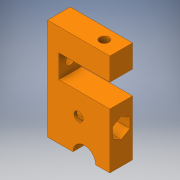
# Autodesk Inventor part: vexOverSupportForArm
Saved by Autodesk Inventor 2016 SP1 (Build 200210100, 210)
## iProperties
Created: 2015-08-15
Part Number: vexOverSupportForArm
Material: Generic
Document SubType Name: Modeling
Designer: steele
Density: 1 g/cm^3
Appearance: Orange
Author: steele
Autodesk Inventor part; units mm, degrees
note: some values were not read from the file. Chosen so that the rebuilt part matches the saved one: direction of "Hole8".
ref_plane "YZ Plane" through (0, 0, 0) normal (1, 0, 0) x (0, 1, 0)
ref_plane "XZ Plane" through (0, 0, 0) normal (0, 1, 0) x (-1, 0, 0)
ref_plane "XY Plane" through (0, 0, 0) normal (0, 0, 1) x (1, 0, 0)
sketch "Sketch1" plane through (0, 0, 0) normal (0, 0, 1) x (1, 0, 0)
  line L0 (0, 0) -> (-34.798, 0)
  line L1 (-34.798, 0) -> (-34.798, -56.642)
  line L2 (0, -12.7) -> (-28.448, -12.7)
  line L3 (-28.448, -12.7) -> (-28.448, -25.654)
  line L4 (-28.448, -25.654) -> (0, -25.654)
  line L5 (0, -56.642) -> (0, -25.654)
  line L6 (0, -12.7) -> (0, 0)
  arc A0 (-7.874, -56.642) -> (-20.574, -56.642) centre (-14.224, -56.642) ccw
  line L7 (-34.798, -56.642) -> (-20.574, -56.642)
  line L8 (-7.874, -56.642) -> (0, -56.642)
  dimension "d0" = 56.642
  dimension "d1" = 34.798
  dimension "d4" = 12.7
  dimension "d5" = 28.448
  dimension "d6" = 12.954
  dimension "d50" = 6.35
  dimension "d51" = 14.224
  dimension "d71" = 56.642
  dimension "d72" = 56.642
  constraints: 18 end point, 4 parallel, 2 horizontal, 2 perpendicular, 2 point on circle, 1 centre point, 1 collinear
  measures "d0" distance of L0.end L1.end
  measures "d1" distance of L0.start L0.end
  measures "d4" distance between parallel lines of L2 L0
  measures "d5" distance of L2.start L2.end
  measures "d6" distance between parallel lines of L4 L2
  measures "d50" radius of A0
  measures "d51" distance from line of A0.centre L5
  measures "d71" distance from line of L0 A0.centre
  measures "d72" distance between parallel lines of L0 L8
extrude "Extrusion4" add sketch "Sketch1" along normal mid plane 12.7
sketch "Sketch9" plane through (-34.798, -56.642, 6.35) normal (-1, 0, 0) x (0, 0, 1)
  line L0 (-12.7, 30.988) -> (0, 30.988) construction
  line L1 (-12.7, 0) -> (-12.7, 6.35) construction
  line L2 (0, 30.988) -> (-12.7, 6.35) construction
  line L3 (0, 6.35) -> (0, 0) construction
  line L4 (0, 6.35) -> (-12.7, 30.988) construction
  line L5 (-6.35, 24.3149) -> (-1.4605, 21.492)
  line L6 (-1.4605, 21.492) -> (-1.4605, 15.846)
  line L7 (-1.4605, 15.846) -> (-6.35, 13.0231)
  line L8 (-6.35, 13.0231) -> (-11.2395, 15.846)
  line L9 (-11.2395, 15.846) -> (-11.2395, 21.492)
  line L10 (-11.2395, 21.492) -> (-6.35, 24.3149)
  line L11 (-12.7, 0) -> (-12.7, 56.642) projected
  point P0 (-6.35, 56.642)
  point P1 (-6.35, 18.669)
  dimension "d61" = 9.779
  constraints: 16 end point, 1 midpoint, 1 parallel, 13 other
  measures "d61" distance between parallel lines of L6 L9
extrude "Extrusion5" cut sketch "Sketch9" against normal through all
sketch "Sketch10" plane through (0, 0, -6.35) normal (0, 0, -1) x (-1, 0, 0)
  line L0 (34.798, -40.796) -> (0, -40.796) projected
  line L1 (34.798, -35.15) -> (0, -35.15) projected
  line L2 (0, -35.15) -> (34.798, -40.796) construction
  line L3 (34.798, -35.15) -> (0, -35.15) construction
  line L4 (0, -40.796) -> (34.798, -35.15) construction
  point P0 (0, 0)
  point P1 (17.399, -37.973)
  constraints: 4 end point, 1 midpoint
hole "Hole6" at (-17.399, -37.973, -6.35) direction (0, 0, 1) diameter 5.1054 end through all clearance for "Flat Head Machine Screw (82)" size "#10" standard "Ansi Unified Screw Threads"
sketch "Sketch11" plane through (-28.448, -25.654, 6.35) normal (1, 0, 0) x (0, 0, -1)
  line L0 (0, -30.988) -> (0, 0) construction
  line L1 (12.7, 12.954) -> (12.7, 0) construction
  line L2 (0, 0) -> (12.7, 12.954) construction
  line L3 (12.7, 12.954) -> (0, 12.954) construction
  line L4 (12.7, 12.954) -> (0, 12.954) construction
  line L5 (0, 12.954) -> (12.7, 0) construction
  point P0 (6.35, 25.654)
  point P1 (6.35, 6.477)
  constraints: 6 end point, 1 collinear, 1 midpoint
hole "Hole7" at (-28.448, -19.177, 0) direction (-1, 0, 0) diameter 5.1054 end through all clearance for "Flat Head Machine Screw (82)" size "#10" standard "Ansi Unified Screw Threads"
sketch "Sketch12" plane through (-34.798, 0, 6.35) normal (0, 1, 0) x (1, 0, 0)
  line L0 (0, 12.7) -> (0, 0) construction
  point P0 (34.798, 6.35)
  point P1 (25.4, 6.35)
  dimension "d80" = 25.4
  measures "d80" distance from line of point (25.4, 6.35) L0
hole "Hole8" at (-9.398, 0, 0) direction (0, -1, 0) diameter 5.1054 end up to surface clearance for "Flat Head Machine Screw (82)" size "#10" standard "Ansi Unified Screw Threads"
equation "\"d6\" = slotWidth + printerOffset"
equation "\"d50\" = 0.5 * outsideCylnderDiam"
equation "\"d51\" = centerLineOfCylinder"
equation "\"d52\" = partWidth"
equation "\"d61\" = hexTubing"
equation "\"d62\" = partWidth"
equation "\"centerLineOfCylinder\" = 14.224"
equation "\"slotWidth\" = 12.7"
equation "\"outsideCylnderDiam\" = 12.7"
equation "\"partWidth\" = 12.7"
equation "\"printerOffset\" = 0.254"
equation "\"hexTubing\" = 9.779"
body "Solid2"
